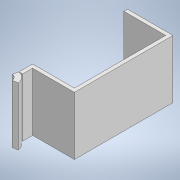
# Autodesk Inventor part: prototype_12_cover
Saved by Autodesk Inventor 2022 (Build 260153000, 153)
## iProperties
Created: 2022-06-23
Part Number: prototype_12_cover
Material: Generic
Document SubType Name: Modeling
Designer: tecware
Density: 1 g/cm^3
Appearance: Default
Author: tecware
Autodesk Inventor part; units mm, degrees
ref_plane "YZ Plane" through (0, 0, 0) normal (1, 0, 0) x (0, 1, 0)
ref_plane "XZ Plane" through (0, 0, 0) normal (0, 1, 0) x (-1, 0, 0)
ref_plane "XY Plane" through (0, 0, 0) normal (0, 0, 1) x (1, 0, 0)
sketch "Sketch1" plane through (0, 0, 0) normal (0, 1, 0) x (-1, 0, 0)
  line L0 (-0.0003, 59.6701) -> (0.6715, 62.594) projected
  line L1 (-2.2, 66.2) -> (-5.2, 66.2) projected
  arc A0 (-2.2, 66.2) -> (0.6715, 62.594) centre (1.5992, 66.279) ccw
  arc A1 (-5.2, 66.2) -> (-0.0003, 59.6701) centre (1.5, 66.2) ccw
  line L2 (-25, 0) -> (0, 0)
  line L3 (0, 19.4) -> (-7, 19.4)
  line L4 (-7, 19.4) -> (-7, 35.6)
  line L5 (-7, 35.6) -> (0, 35.6)
  line L6 (-0.0003, 59.6701) -> (-0.0002, 52.1701)
  line L7 (-0.0003, 59.6701) -> (-2.0003, 59.6701)
  line L8 (-2.0003, 59.6701) -> (-2.0003, 52.1701)
  line L9 (-2.0003, 52.1701) -> (-0.0002, 52.1701)
  line L10 (-2.0003, 52.1701) -> (-25, 52.1701)
  line L11 (-25, 52.1701) -> (-25, 54.1701)
  line L12 (-25, 54.1701) -> (-2.0003, 54.1701)
  line L13 (-2.0003, 54.1701) -> (-2.0003, 52.1701)
  line L14 (-2.0003, 59.6701) -> (-3.8832, 62.2111)
  line L15 (-25, 52.1701) -> (-23, 52.1701)
  line L16 (-23, 52.1701) -> (-23, 0)
  line L17 (-23, 0) -> (-25, 0)
  line L18 (-25, 0) -> (-25, 52.1701)
  line L19 (0, 0) -> (-23, 0)
  line L20 (-23, 0) -> (-23, 2)
  line L21 (-23, 2) -> (0, 2)
  line L22 (0, 2) -> (0, 0)
  point P0 (-2.0003, 54.1701)
  dimension "d0" = 3.8
  dimension "d1" = 6.7
  dimension "d2" = 7.5
  dimension "d3" = 2
  dimension "d4" = 2
  dimension "d5" = 2
  dimension "d6" = 2
  constraints: 42 end point, 5 point on circle, 2 centre point, 2 point on line, 3 other
  measures "d0" radius of A0
  measures "d1" radius of A1
  measures "d2" distance of L0.start L6.end
  measures "d3" distance of L0.start L7.end
  measures "d4" distance of L10.end L11.end
  measures "d5" distance of L16.end L17.end
  measures "d6" distance of L19.end L20.end
extrude "Extrusion1" add sketch "Sketch1" along normal mid plane 32 contours A1 L1 A0 L0 | L7 L14 A1 | L6 L9 L8 L7 | L10 L11 L12 L8 | L16 L2 L18 L10
body "Solid1"
